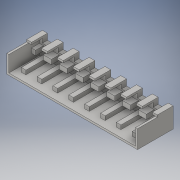
# Autodesk Inventor part: EndcapWithSlotholes
Saved by Autodesk Inventor 2016 (Build 200138000, 138)
## iProperties
Created: 2016-03-27
Part Number: EndcapWithSlotholes
Material: Generic
Document SubType Name: Modeling
Designer: Scott
Density: 1 g/cm^3
Appearance: Default
Author: Scott
Autodesk Inventor part; units mm, degrees
ref_plane "YZ Plane" through (0, 0, 0) normal (1, 0, 0) x (0, 1, 0)
ref_plane "XZ Plane" through (0, 0, 0) normal (0, 1, 0) x (-1, 0, 0)
ref_plane "XY Plane" through (0, 0, 0) normal (0, 0, 1) x (1, 0, 0)
sketch "Sketch1" plane through (0, 0, 0) normal (0, 0, 1) x (1, 0, 0)
  line L0 (80, -10.16) -> (-80, -10.16)
  line L1 (-80, -10.16) -> (-80, 10.16)
  line L2 (-80, 10.16) -> (80, 10.16)
  line L3 (80, 10.16) -> (80, -10.16)
  line L4 (80, -10.16) -> (-80, 10.16) construction
  line L5 (-80, -10.16) -> (80, 10.16) construction
  line L6 (-85.08, -2.921) -> (-74.92, -2.921)
  line L7 (-74.92, -2.921) -> (-74.92, 2.921)
  line L8 (-74.92, 2.921) -> (-85.08, 2.921)
  line L9 (-85.08, 2.921) -> (-85.08, -2.921)
  line L10 (-85.08, -2.921) -> (-74.92, 2.921) construction
  line L11 (-74.92, -2.921) -> (-85.08, 2.921) construction
  point P0 (0, 0)
  point P1 (-80, 0)
  dimension "d0" = 160
  dimension "d1" = 20.32
  dimension "d2" = 10.16
  dimension "d3" = 5.842
  constraints: 24 end point, 5 midpoint, 4 parallel, 2 horizontal, 2 perpendicular
  measures "d0" distance of L1.end L2.end
  measures "d1" distance of L0.end L1.end
  measures "d2" distance of L8.end L7.end
  measures "d3" distance of L7.end L6.end
extrude "Extrusion1" add sketch "Sketch1" along normal blind 6.35 contours L0 L1 L6 L7 L8 L2 L3 | L1 L8 L7 L6
sketch "Sketch2" plane through (0, 0, 6.35) normal (0, 0, 1) x (1, 0, 0)
  line L0 (-74.92, -2.921) -> (-80, -2.921)
  line L1 (-80, 2.921) -> (-74.92, 2.921)
  line L2 (-74.92, 2.921) -> (-74.92, -2.921)
  line L3 (-80, 10.16) -> (-80, -10.16) projected
  line L4 (-80, 0) -> (-70, 0)
  line L5 (-80, 2.921) -> (-80, -2.921)
  line L6 (-67.079, -4.92) -> (-67.079, -10)
  line L7 (-72.921, -10) -> (-72.921, -4.92)
  line L8 (-72.921, -4.92) -> (-67.079, -4.92)
  line L9 (-72.921, -10) -> (-67.079, -10)
  line L10 (-65.08, 2.921) -> (-60, 2.921)
  line L11 (-60, -2.921) -> (-65.08, -2.921)
  line L12 (-65.08, -2.921) -> (-65.08, 2.921)
  line L13 (-60, -2.921) -> (-60, 2.921)
  line L14 (-72.921, 4.92) -> (-72.921, 10)
  line L15 (-67.079, 10) -> (-67.079, 4.92)
  line L16 (-67.079, 4.92) -> (-72.921, 4.92)
  line L17 (-67.079, 10) -> (-72.921, 10)
  line L18 (-45.08, -2.921) -> (-45.08, 2.921)
  line L19 (-40, -2.921) -> (-45.08, -2.921)
  line L20 (-40, -2.921) -> (-40, 2.921)
  line L21 (-45.08, 2.921) -> (-40, 2.921)
  line L22 (-47.079, 4.92) -> (-52.921, 4.92)
  line L23 (-52.921, 4.92) -> (-52.921, 10)
  line L24 (-47.079, 10) -> (-52.921, 10)
  line L25 (-47.079, 10) -> (-47.079, 4.92)
  line L26 (-54.92, -2.921) -> (-60, -2.921)
  line L27 (-60, 2.921) -> (-54.92, 2.921)
  line L28 (-54.92, 2.921) -> (-54.92, -2.921)
  line L29 (-60, 2.921) -> (-60, -2.921)
  line L30 (-60, 0) -> (-50, 0)
  line L31 (-47.079, -4.92) -> (-47.079, -10)
  line L32 (-52.921, -10) -> (-52.921, -4.92)
  line L33 (-52.921, -10) -> (-47.079, -10)
  line L34 (-52.921, -4.92) -> (-47.079, -4.92)
  line L35 (-25.08, -2.921) -> (-25.08, 2.921)
  line L36 (-20, -2.921) -> (-25.08, -2.921)
  line L37 (-20, -2.921) -> (-20, 2.921)
  line L38 (-25.08, 2.921) -> (-20, 2.921)
  line L39 (-27.079, 4.92) -> (-32.921, 4.92)
  line L40 (-32.921, 4.92) -> (-32.921, 10)
  line L41 (-27.079, 10) -> (-32.921, 10)
  line L42 (-27.079, 10) -> (-27.079, 4.92)
  line L43 (-34.92, -2.921) -> (-40, -2.921)
  line L44 (-40, 2.921) -> (-34.92, 2.921)
  line L45 (-34.92, 2.921) -> (-34.92, -2.921)
  line L46 (-40, 2.921) -> (-40, -2.921)
  line L47 (-40, 0) -> (-30, 0)
  line L48 (-27.079, -4.92) -> (-27.079, -10)
  line L49 (-32.921, -10) -> (-32.921, -4.92)
  line L50 (-32.921, -10) -> (-27.079, -10)
  line L51 (-32.921, -4.92) -> (-27.079, -4.92)
  line L52 (-5.08, -2.921) -> (-5.08, 2.921)
  line L53 (0, -2.921) -> (-5.08, -2.921)
  line L54 (0, -2.921) -> (0, 2.921)
  line L55 (-5.08, 2.921) -> (0, 2.921)
  line L56 (-7.079, 4.92) -> (-12.921, 4.92)
  line L57 (-12.921, 4.92) -> (-12.921, 10)
  line L58 (-7.079, 10) -> (-12.921, 10)
  line L59 (-7.079, 10) -> (-7.079, 4.92)
  line L60 (-14.92, -2.921) -> (-20, -2.921)
  line L61 (-20, 2.921) -> (-14.92, 2.921)
  line L62 (-14.92, 2.921) -> (-14.92, -2.921)
  line L63 (-20, 2.921) -> (-20, -2.921)
  line L64 (-20, 0) -> (-10, 0)
  line L65 (-7.079, -4.92) -> (-7.079, -10)
  line L66 (-12.921, -10) -> (-12.921, -4.92)
  line L67 (-12.921, -10) -> (-7.079, -10)
  line L68 (-12.921, -4.92) -> (-7.079, -4.92)
  line L69 (14.92, -2.921) -> (14.92, 2.921)
  line L70 (20, -2.921) -> (14.92, -2.921)
  line L71 (20, -2.921) -> (20, 2.921)
  line L72 (14.92, 2.921) -> (20, 2.921)
  line L73 (12.921, 4.92) -> (7.079, 4.92)
  line L74 (7.079, 4.92) -> (7.079, 10)
  line L75 (12.921, 10) -> (7.079, 10)
  line L76 (12.921, 10) -> (12.921, 4.92)
  line L77 (5.08, -2.921) -> (0, -2.921)
  line L78 (0, 2.921) -> (5.08, 2.921)
  line L79 (5.08, 2.921) -> (5.08, -2.921)
  line L80 (0, 2.921) -> (0, -2.921)
  line L81 (0, 0) -> (10, 0)
  line L82 (12.921, -4.92) -> (12.921, -10)
  line L83 (7.079, -10) -> (7.079, -4.92)
  line L84 (7.079, -10) -> (12.921, -10)
  line L85 (7.079, -4.92) -> (12.921, -4.92)
  line L86 (34.92, -2.921) -> (34.92, 2.921)
  line L87 (40, -2.921) -> (34.92, -2.921)
  line L88 (40, -2.921) -> (40, 2.921)
  line L89 (34.92, 2.921) -> (40, 2.921)
  line L90 (32.921, 4.92) -> (27.079, 4.92)
  line L91 (27.079, 4.92) -> (27.079, 10)
  line L92 (32.921, 10) -> (27.079, 10)
  line L93 (32.921, 10) -> (32.921, 4.92)
  line L94 (25.08, -2.921) -> (20, -2.921)
  line L95 (20, 2.921) -> (25.08, 2.921)
  line L96 (25.08, 2.921) -> (25.08, -2.921)
  line L97 (20, 2.921) -> (20, -2.921)
  line L98 (20, 0) -> (30, 0)
  line L99 (32.921, -4.92) -> (32.921, -10)
  line L100 (27.079, -10) -> (27.079, -4.92)
  line L101 (27.079, -10) -> (32.921, -10)
  line L102 (27.079, -4.92) -> (32.921, -4.92)
  line L103 (54.92, -2.921) -> (54.92, 2.921)
  line L104 (60, -2.921) -> (54.92, -2.921)
  line L105 (60, -2.921) -> (60, 2.921)
  line L106 (54.92, 2.921) -> (60, 2.921)
  line L107 (52.921, 4.92) -> (47.079, 4.92)
  line L108 (47.079, 4.92) -> (47.079, 10)
  line L109 (52.921, 10) -> (47.079, 10)
  line L110 (52.921, 10) -> (52.921, 4.92)
  line L111 (45.08, -2.921) -> (40, -2.921)
  line L112 (40, 2.921) -> (45.08, 2.921)
  line L113 (45.08, 2.921) -> (45.08, -2.921)
  line L114 (40, 2.921) -> (40, -2.921)
  line L115 (40, 0) -> (50, 0)
  line L116 (52.921, -4.92) -> (52.921, -10)
  line L117 (47.079, -10) -> (47.079, -4.92)
  line L118 (47.079, -10) -> (52.921, -10)
  line L119 (47.079, -4.92) -> (52.921, -4.92)
  line L120 (74.92, -2.921) -> (74.92, 2.921)
  line L121 (80, -2.921) -> (74.92, -2.921)
  line L122 (80, -2.921) -> (80, 2.921)
  line L123 (74.92, 2.921) -> (80, 2.921)
  line L124 (72.921, 4.92) -> (67.079, 4.92)
  line L125 (67.079, 4.92) -> (67.079, 10)
  line L126 (72.921, 10) -> (67.079, 10)
  line L127 (72.921, 10) -> (72.921, 4.92)
  line L128 (65.08, -2.921) -> (60, -2.921)
  line L129 (60, 2.921) -> (65.08, 2.921)
  line L130 (65.08, 2.921) -> (65.08, -2.921)
  line L131 (60, 2.921) -> (60, -2.921)
  line L132 (60, 0) -> (70, 0)
  line L133 (72.921, -4.92) -> (72.921, -10)
  line L134 (67.079, -10) -> (67.079, -4.92)
  line L135 (67.079, -10) -> (72.921, -10)
  line L136 (67.079, -4.92) -> (72.921, -4.92)
  point P0 (0, 0)
  point P1 (-70, -10)
  point P2 (-60, 0)
  point P3 (-70, 10)
  point P4 (-40, 0)
  point P5 (-50, 10)
  point P6 (-60, 10.16)
  point P7 (-60, -10.16)
  point P8 (-50, -10)
  point P9 (-20, 0)
  point P10 (-30, 10)
  point P11 (-40, 10.16)
  point P12 (-40, -10.16)
  point P13 (-30, -10)
  point P14 (0, 0)
  point P15 (-10, 10)
  point P16 (-20, 10.16)
  point P17 (-20, -10.16)
  point P18 (-10, -10)
  point P19 (20, 0)
  point P20 (10, 10)
  point P21 (0, 10.16)
  point P22 (0, -10.16)
  point P23 (10, -10)
  point P24 (40, 0)
  point P25 (30, 10)
  point P26 (20, 10.16)
  point P27 (20, -10.16)
  point P28 (30, -10)
  point P29 (60, 0)
  point P30 (50, 10)
  point P31 (40, 10.16)
  point P32 (40, -10.16)
  point P33 (50, -10)
  point P34 (80, 0)
  point P35 (70, 10)
  point P36 (60, 10.16)
  point P37 (60, -10.16)
  point P38 (70, -10)
  dimension "d8" = 10
  dimension "d11" = 360
  dimension "d15" = 20
  constraints: 272 end point, 3 horizontal, 2 point on line, 1 collinear, 1 midpoint, 1 parallel, 1 vertical, 316 other
  measures "d8" distance of L4.start L4.end
  measures "d15" distance of L4.end L30.end
extrude "Extrusion2" add sketch "Sketch2" along normal blind 10
sketch "Sketch3" plane through (0, 0, 6.35) normal (0, 0, 1) x (1, 0, 0)
  point P0 (0, 0)
sketch "Sketch4" plane through (0, 0, 0) normal (0, 0, -1) x (-1, 0, 0)
  line L0 (-80, -10.16) -> (80, -10.16) projected
  line L1 (80, -10.16) -> (80, 10.16) projected
  line L2 (80, 10.16) -> (-80, 10.16) projected
  line L3 (-80, 10.16) -> (-80, -10.16) projected
  line L4 (82.54, 12.7) -> (82.54, -12.7)
  line L5 (82.54, -12.7) -> (-82.54, -12.7)
  line L6 (-82.54, -12.7) -> (-82.54, 12.7)
  line L7 (-82.54, 12.7) -> (82.54, 12.7)
  point P0 (0, 0)
  dimension "d22" = 2.54
  constraints: 8 end point, 3 other
  measures "d22" distance between parallel lines of L1 L4
extrude "Extrusion3" add sketch "Sketch4" against normal blind 20
sketch "Sketch5" plane through (0, 0, 20) normal (0, 0, 1) x (1, 0, 0)
  line L0 (-80, -10.16) -> (-80, 10.16) projected
  line L1 (-80, 10.16) -> (80, 10.16) projected
  line L2 (80, 10.16) -> (80, -10.16) projected
  line L3 (80, -10.16) -> (-80, -10.16) projected
  line L4 (-82.54, 12.7) -> (-82.54, -12.7) projected
  line L5 (-82.54, -12.7) -> (82.54, -12.7) projected
  line L6 (82.54, -12.7) -> (82.54, 12.7) projected
  line L7 (82.54, 12.7) -> (-82.54, 12.7) projected
  line L8 (80, 10.16) -> (-80, 10.16) projected
  line L9 (-80, 10.16) -> (-82.54, 10.16)
  line L10 (80, 10.16) -> (82.54, 10.16)
  line L11 (82.54, -12.7) -> (82.54, 12.7) projected
  point P0 (0, 0)
  constraints: 4 end point, 3 point on line, 1 perpendicular
extrude "Extrusion4" add sketch "Sketch5" along normal blind 25 contours L3 L2 L10 L6 L5 L4 L9 L0
sketch "Sketch6" plane through (0, 0, 16.35) normal (0, 0, 1) x (1, 0, 0)
  line L0 (-67.079, -10) -> (-67.079, -4.92) projected
  line L1 (-67.079, -4.92) -> (-72.921, -4.92) projected
  line L2 (-72.921, -4.92) -> (-72.921, -10) projected
  line L3 (-72.921, -10) -> (-67.079, -10) projected
  line L4 (-47.079, -10) -> (-47.079, -4.92) projected
  line L5 (-47.079, -4.92) -> (-52.921, -4.92) projected
  line L6 (-52.921, -4.92) -> (-52.921, -10) projected
  line L7 (-52.921, -10) -> (-47.079, -10) projected
  line L8 (-27.079, -10) -> (-27.079, -4.92) projected
  line L9 (-27.079, -4.92) -> (-32.921, -4.92) projected
  line L10 (-32.921, -4.92) -> (-32.921, -10) projected
  line L11 (-32.921, -10) -> (-27.079, -10) projected
  line L12 (-7.079, -10) -> (-7.079, -4.92) projected
  line L13 (-7.079, -4.92) -> (-12.921, -4.92) projected
  line L14 (-12.921, -4.92) -> (-12.921, -10) projected
  line L15 (-12.921, -10) -> (-7.079, -10) projected
  line L16 (12.921, -10) -> (12.921, -4.92) projected
  line L17 (12.921, -4.92) -> (7.079, -4.92) projected
  line L18 (7.079, -4.92) -> (7.079, -10) projected
  line L19 (7.079, -10) -> (12.921, -10) projected
  line L20 (32.921, -10) -> (32.921, -4.92) projected
  line L21 (32.921, -4.92) -> (27.079, -4.92) projected
  line L22 (27.079, -4.92) -> (27.079, -10) projected
  line L23 (27.079, -10) -> (32.921, -10) projected
  line L24 (52.921, -10) -> (52.921, -4.92) projected
  line L25 (52.921, -4.92) -> (47.079, -4.92) projected
  line L26 (47.079, -4.92) -> (47.079, -10) projected
  line L27 (47.079, -10) -> (52.921, -10) projected
  line L28 (72.921, -10) -> (72.921, -4.92) projected
  line L29 (72.921, -4.92) -> (67.079, -4.92) projected
  line L30 (67.079, -4.92) -> (67.079, -10) projected
  line L31 (67.079, -10) -> (72.921, -10) projected
  point P0 (0, 0)
extrude "Extrusion5" add sketch "Sketch6" along normal blind 20
sketch "Sketch7" plane through (0, 0, 16.35) normal (0, 0, 1) x (1, 0, 0)
  line L0 (-72.921, 10) -> (-72.921, 4.92) projected
  line L1 (-72.921, 4.92) -> (-67.079, 4.92) projected
  line L2 (-67.079, 4.92) -> (-67.079, 10) projected
  line L3 (-67.079, 10) -> (-72.921, 10) projected
  line L4 (-67.079, 4.92) -> (-72.921, 4.92) projected
  line L5 (-70, 4.92) -> (-63.65, 4.92)
  line L6 (-63.65, 4.92) -> (-63.65, 17.9959)
  line L7 (-63.65, 17.9959) -> (-76.35, 17.9959)
  line L8 (-76.35, 17.9959) -> (-76.35, 4.92)
  line L9 (-76.35, 4.92) -> (-70, 4.92)
  line L10 (-50, 4.92) -> (-43.65, 4.92)
  line L11 (-43.65, 4.92) -> (-43.65, 17.9959)
  line L12 (-43.65, 17.9959) -> (-56.35, 17.9959)
  line L13 (-56.35, 17.9959) -> (-56.35, 4.92)
  line L14 (-56.35, 4.92) -> (-50, 4.92)
  line L15 (-30, 4.92) -> (-23.65, 4.92)
  line L16 (-23.65, 4.92) -> (-23.65, 17.9959)
  line L17 (-23.65, 17.9959) -> (-36.35, 17.9959)
  line L18 (-36.35, 17.9959) -> (-36.35, 4.92)
  line L19 (-36.35, 4.92) -> (-30, 4.92)
  line L20 (-10, 4.92) -> (-3.65, 4.92)
  line L21 (-3.65, 4.92) -> (-3.65, 17.9959)
  line L22 (-3.65, 17.9959) -> (-16.35, 17.9959)
  line L23 (-16.35, 17.9959) -> (-16.35, 4.92)
  line L24 (-16.35, 4.92) -> (-10, 4.92)
  line L25 (10, 4.92) -> (16.35, 4.92)
  line L26 (16.35, 4.92) -> (16.35, 17.9959)
  line L27 (16.35, 17.9959) -> (3.65, 17.9959)
  line L28 (3.65, 17.9959) -> (3.65, 4.92)
  line L29 (3.65, 4.92) -> (10, 4.92)
  line L30 (30, 4.92) -> (36.35, 4.92)
  line L31 (36.35, 4.92) -> (36.35, 17.9959)
  line L32 (36.35, 17.9959) -> (23.65, 17.9959)
  line L33 (23.65, 17.9959) -> (23.65, 4.92)
  line L34 (23.65, 4.92) -> (30, 4.92)
  line L35 (50, 4.92) -> (56.35, 4.92)
  line L36 (56.35, 4.92) -> (56.35, 17.9959)
  line L37 (56.35, 17.9959) -> (43.65, 17.9959)
  line L38 (43.65, 17.9959) -> (43.65, 4.92)
  line L39 (43.65, 4.92) -> (50, 4.92)
  line L40 (70, 4.92) -> (76.35, 4.92)
  line L41 (76.35, 4.92) -> (76.35, 17.9959)
  line L42 (76.35, 17.9959) -> (63.65, 17.9959)
  line L43 (63.65, 17.9959) -> (63.65, 4.92)
  line L44 (63.65, 4.92) -> (70, 4.92)
  point P0 (0, 0)
  dimension "d29" = 6.35
  dimension "d30" = 12.7
  dimension "d33" = 20
  constraints: 80 end point, 8 point on line, 4 perpendicular, 2 horizontal, 1 collinear, 1 midpoint, 69 other
  measures "d29" distance of L5.start L5.end
  measures "d30" distance of L6.end L7.end
  measures "d33" distance of L5.start L10.start
extrude "Extrusion6" cut sketch "Sketch7" along normal mid plane 76.2
body "Solid1"
